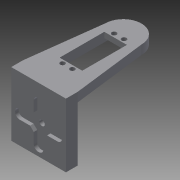
# Autodesk Inventor part: FrontUpperLegShoulder
Saved by Autodesk Inventor 2014 SP1 (Build 180222100, 222)
## iProperties
Created: 2013-09-20
Part Number: FrontUpperLegShoulder
Material: Generic
Document SubType Name: Modeling
Designer: Medrimonia
Density: 1 g/cm^3
Appearance: Default
FrontUpperLegShoulderWidth: 30,000 mm
Author: Medrimonia
Autodesk Inventor part; units mm, degrees
ref_plane "YZ Plane" through (0, 0, 0) normal (1, 0, 0) x (0, 1, 0)
ref_plane "XZ Plane" through (0, 0, 0) normal (0, 1, 0) x (-1, 0, 0)
ref_plane "XY Plane" through (0, 0, 0) normal (0, 0, 1) x (1, 0, 0)
sketch "Sketch1" plane through (0, 0, 0) normal (0, 1, 0) x (-1, 0, 0)
  line L0 (-15, -15) -> (15, -15)
  line L1 (15, -15) -> (15, 15)
  line L2 (15, 15) -> (-15, 15)
  line L3 (-15, 15) -> (-15, -15)
  line L4 (-15, -15) -> (15, 15) construction
  line L5 (15, -15) -> (-15, 15) construction
  line L6 (-2.45, -12.65) -> (2.45, -12.65) construction
  line L7 (2.45, -12.65) -> (2.45, 12.65) construction
  line L8 (2.45, 12.65) -> (-2.45, 12.65) construction
  line L9 (-2.45, 12.65) -> (-2.45, -12.65) construction
  line L10 (-2.45, -12.65) -> (2.45, 12.65) construction
  line L11 (2.45, -12.65) -> (-2.45, 12.65) construction
  line L12 (-12.65, -2.45) -> (12.65, -2.45) construction
  line L13 (12.65, -2.45) -> (12.65, 2.45) construction
  line L14 (12.65, 2.45) -> (-12.65, 2.45) construction
  line L15 (-12.65, 2.45) -> (-12.65, -2.45) construction
  line L16 (-12.65, -2.45) -> (12.65, 2.45) construction
  line L17 (12.65, -2.45) -> (-12.65, 2.45) construction
  line L18 (-12.85, -2.65) -> (12.85, -2.65)
  line L19 (12.85, -2.65) -> (12.85, 2.65)
  line L20 (12.85, 2.65) -> (-12.85, 2.65)
  line L21 (-12.85, 2.65) -> (-12.85, -2.65)
  line L22 (-12.85, -2.65) -> (12.85, 2.65) construction
  line L23 (12.85, -2.65) -> (-12.85, 2.65) construction
  line L24 (-2.65, -12.85) -> (2.65, -12.85)
  line L25 (2.65, -12.85) -> (2.65, 12.85)
  line L26 (2.65, 12.85) -> (-2.65, 12.85)
  line L27 (-2.65, 12.85) -> (-2.65, -12.85)
  line L28 (-2.65, -12.85) -> (2.65, 12.85) construction
  line L29 (2.65, -12.85) -> (-2.65, 12.85) construction
  point P0 (0, 0)
  point P1 (0, 0)
  dimension "d0" = 30
  dimension "d1" = 4.9
  dimension "d2" = 10.2
  dimension "d3" = 0.2
  dimension "d4" = 0.2
  constraints: 60 end point, 12 midpoint, 10 parallel, 10 perpendicular, 5 horizontal
  measures "d0" distance of L1.end L2.end
  measures "d1" distance of L14.end L12.start
  measures "d2" distance between parallel lines of L13 L7
  measures "d3" distance between parallel lines of L25 L7
  measures "d4" distance between parallel lines of L26 L8
extrude "Extrusion1" add sketch "Sketch1" along normal blind 1.9
sketch "Sketch2" plane through (0, 1.9, 0) normal (0, 1, 0) x (1, 0, 0)
  line L0 (15, 15) -> (-15, 15) projected
  line L1 (-15, 15) -> (-15, -15) projected
  line L2 (-15, -15) -> (15, -15) projected
  line L3 (15, -15) -> (15, 15) projected
  circle A0 centre (0, 0) radius 1.5
  dimension "d7" = 3
  constraints: 1 centre point, 1 coincident
  measures "d7" diameter of A0
extrude "Extrusion2" add sketch "Sketch2" along normal blind 2
sketch "Sketch3" plane through (0, 3.9, 0) normal (0, 1, 0) x (1, 0, 0)
  circle A0 centre (0, 0) radius 1.5 projected
  line L0 (15, 15) -> (-15, 15) projected
  line L1 (-15, 15) -> (-15, -15) projected
  line L2 (-15, -15) -> (15, -15) projected
  line L3 (15, -15) -> (15, 15) projected
  circle A1 centre (0, 0) radius 2.75
  dimension "d10" = 5.5
  constraints: 1 centre point, 1 coincident
  measures "d10" diameter of A1
extrude "Extrusion3" add sketch "Sketch3" along normal blind 2.5 contours L3 L2 L1 L0
chamfer "Chamfer1" distance 2 angle 45 1 edges at (-2.65, 0.95, -2.65)
fillet "Fillet1" radius 2.45 1 edges at (-12.85, 0.95, -2.65)
fillet "Fillet2" radius 2.45 1 edges at (-2.65, 0.95, -12.85)
chamfer "Chamfer2" distance 2 angle 45 1 edges at (2.65, 0.95, -2.65)
chamfer "Chamfer3" distance 2 angle 45 1 edges at (2.65, 0.95, 2.65)
fillet "Fillet3" radius 2.45 1 edges at (12.85, 0.95, -2.65)
fillet "Fillet4" radius 2.45 1 edges at (2.65, 0.95, -12.85)
fillet "Fillet5" radius 2.45 1 edges at (12.85, 0.95, 2.65)
fillet "Fillet6" radius 2.45 1 edges at (2.65, 0.95, 12.85)
chamfer "Chamfer4" distance 2 angle 45 1 edges at (-2.65, 0.95, 2.65)
fillet "Fillet7" radius 2.45 2 edges at (-2.65, 0.95, 12.85) (-12.85, 0.95, 2.65)
sketch "Sketch8" plane through (-15, 0, 15) normal (0, 0, 1) x (1, 0, 0)
  line L0 (0, 0) -> (30, 0) projected
  line L1 (30, 0) -> (30, 6.4) projected
  line L2 (0, 6.4) -> (30, 6.4) projected
  line L3 (0, 0) -> (0, 6.4) projected
  line L4 (15, 0) -> (15, 120) construction
  line L5 (30, 6.4) -> (25, 46.4)
  line L6 (25, 46.4) -> (5, 46.4)
  line L7 (5, 46.4) -> (0, 6.4)
  arc A0 (25, 46.4) -> (5, 46.4) centre (15, 46.4) ccw
  dimension "d101" = 40
  dimension "d102" = 20
  constraints: 8 end point, 2 point on circle, 1 centre point, 1 midpoint, 1 perpendicular, 1 other
  measures "d101" distance between parallel lines of L2 L6
  measures "d102" distance of L5.end L6.end
extrude "Extrusion7" add sketch "Sketch8" along normal blind 5
sketch "Sketch9" plane through (-15, 0, 20) normal (0, 0, 1) x (1, 0, 0)
  line L0 (0, 0) -> (30, 0) projected
  line L1 (9.3, 41.75) -> (20.7, 41.75) construction
  line L2 (20.7, 41.75) -> (20.7, 18.25) construction
  line L3 (20.7, 18.25) -> (9.3, 18.25) construction
  line L4 (9.3, 18.25) -> (9.3, 41.75) construction
  line L5 (15, 90) -> (15, 15.8225) construction
  line L6 (9.3, 41.75) -> (9.3, 46.15) construction
  line L7 (9.3, 46.15) -> (20.7, 46.15) construction
  line L8 (20.7, 46.15) -> (20.7, 41.75) construction
  line L9 (20.7, 18.25) -> (20.7, 13.85) construction
  line L10 (20.7, 13.85) -> (9.3, 13.85) construction
  line L11 (9.3, 13.85) -> (9.3, 18.25) construction
  circle A0 centre (12.3, 44.15) radius 1.3
  circle A1 centre (17.7, 44.15) radius 1.3
  line L12 (-17.4512, 30) -> (18.2205, 30) construction
  circle A2 centre (12.3, 15.85) radius 1.3
  circle A3 centre (17.7, 15.85) radius 1.3
  line L13 (8.8, 42.25) -> (21.2, 42.25)
  line L14 (21.2, 42.25) -> (21.2, 17.75)
  line L15 (21.2, 17.75) -> (8.8, 17.75)
  line L16 (8.8, 17.75) -> (8.8, 42.25)
  line L17 (15, 0) -> (15, 83.8502) construction
  dimension "d105" = 11.4
  dimension "d106" = 23.5
  dimension "d107" = 3
  dimension "d108" = 2.4
  dimension "d109" = 4.4
  dimension "d110" = 0.5
  dimension "d111" = 0.5
  dimension "d113" = 2.6
  dimension "d122" = 30
  constraints: 34 end point, 8 parallel, 5 perpendicular, 4 centre point, 3 symmetric about line, 2 collinear, 2 horizontal, 1 point on line, 8 other
  measures "d105" distance between parallel lines of L2 L4
  measures "d106" distance between parallel lines of L3 L1
  measures "d107" distance from line of L6 A0.centre
  measures "d108" distance from line of A3.centre L3
  measures "d109" distance between parallel lines of L1 L7
  measures "d110" distance between parallel lines of L1 L13
  measures "d111" distance between parallel lines of L2 L14
  measures "d113" diameter of A1
  measures "d122" distance between parallel lines of L0 L12
extrude "Extrusion8" cut sketch "Sketch9" against normal through all
sketch "Sketch10" plane through (-15, 0, 20) normal (0, 0, 1) x (1, 0, 0)
  circle A0 centre (17.7, 15.85) radius 1.3 projected
  circle A1 centre (17.7, 44.15) radius 1.3 projected
  circle A2 centre (12.3, 44.15) radius 1.3 projected
  circle A3 centre (12.3, 15.85) radius 1.3 projected
  line L0 (8.8, 17.75) -> (8.8, 42.25) projected
  line L1 (8.8, 42.25) -> (21.2, 42.25) projected
  line L2 (21.2, 42.25) -> (21.2, 17.75) projected
  line L3 (21.2, 17.75) -> (8.8, 17.75) projected
  line L4 (0, 0) -> (30, 0) projected
  line L5 (9.3, 41.75) -> (20.7, 41.75) construction
  line L6 (20.7, 41.75) -> (20.7, 18.25) construction
  line L7 (20.7, 18.25) -> (9.3, 18.25) construction
  line L8 (9.3, 18.25) -> (9.3, 41.75) construction
  line L9 (15, 87.388) -> (15, -76.2197) construction
  line L10 (9.3, 41.75) -> (9.3, 46.15) construction
  line L11 (9.3, 46.15) -> (20.7, 46.15) construction
  line L12 (20.7, 46.15) -> (20.7, 41.75) construction
  line L13 (20.7, 18.25) -> (20.7, 13.85) construction
  line L14 (20.7, 13.85) -> (9.3, 13.85) construction
  line L15 (9.3, 13.85) -> (9.3, 18.25) construction
  line L16 (0.832, 30) -> (29.7617, 30) construction
  line L17 (8.8, 46.65) -> (21.2, 46.65)
  line L18 (21.2, 46.65) -> (21.2, 13.35)
  line L19 (21.2, 13.35) -> (8.8, 13.35)
  line L20 (8.8, 13.35) -> (8.8, 46.65)
  line L21 (15, 0) -> (15, 87.4766) construction
  dimension "d125" = 11.4
  dimension "d126" = 23.5
  dimension "d127" = 4.4
  dimension "d128" = 0.5
  dimension "d130" = 0.5
  dimension "d136" = 30
  constraints: 34 end point, 10 parallel, 5 perpendicular, 2 collinear, 2 horizontal, 1 coincident, 5 other
  measures "d125" distance between parallel lines of L6 L8
  measures "d126" distance between parallel lines of L7 L5
  measures "d127" distance between parallel lines of L5 L11
  measures "d128" distance between parallel lines of L6 L18
  measures "d130" distance between parallel lines of L11 L17
  measures "d136" distance between parallel lines of L4 L16
ref_plane "Work Plane2" through (-15, 0, 17) normal (0, 0, 1) x (1, 0, 0)
extrude "Extrusion10" cut sketch "Sketch10" along normal up to surface (2 mm away) from surface at -5 contours L3 L18 L19 L20 | L20 L17 L18 L1
equation "\"d0\" = FrontUpperLegShoulderWidth"
equation "\"d1\" = ServoArmWidth"
equation "\"d2\" = ServoArmLength"
equation "\"d3\" = ServoArmSpacing"
equation "\"d4\" = ServoArmSpacing"
equation "\"d5\" = ServoArmThickness"
equation "\"d7\" = ServoArmHoleRequired"
equation "\"d8\" = MinimalThickness"
equation "\"d10\" = ServoArmHeadScrewTrace"
equation "\"d11\" = ServoArmHeadScrewThickness"
equation "\"d13\" = ServoArmInternFillet"
equation "\"d16\" = ServoArmExternFillet"
equation "\"d17\" = ServoArmExternFillet"
equation "\"d18\" = ServoArmInternFillet"
equation "\"d21\" = ServoArmInternFillet"
equation "\"d24\" = ServoArmExternFillet"
equation "\"d25\" = ServoArmExternFillet"
equation "\"d26\" = ServoArmExternFillet"
equation "\"d27\" = ServoArmExternFillet"
equation "\"d28\" = ServoArmInternFillet"
equation "\"d31\" = ServoArmExternFillet"
equation "\"d101\" = FrontShoulderHeight"
equation "\"d102\" = FrontShoulderWidth"
equation "\"d103\" = FrontShoulderThickness"
equation "\"d105\" = ServoCoreWidth"
equation "\"d106\" = ServoCoreLength"
equation "\"d107\" = ServoEdgeToFixation"
equation "\"d108\" = ServoCoreToFixation"
equation "\"d109\" = ServoFixationLength"
equation "\"d110\" = ServoTraceSpacing"
equation "\"d111\" = ServoTraceSpacing"
equation "\"d113\" = ServoScrewDiameterRequired"
equation "\"d122\" = FrontShoulderServoCenterDistance"
equation "\"d123\" = FrontShoulderThickness"
equation "\"d125\" = ServoCoreWidth"
equation "\"d126\" = ServoCoreLength"
equation "\"d127\" = ServoFixationLength"
equation "\"d128\" = ServoTraceSpacing"
equation "\"d130\" = ServoTraceSpacing"
equation "\"d136\" = FrontShoulderServoCenterDistance"
equation "\"ServoTraceSpacing\" = 0.5"
equation "\"FrontUpperLegShoulderWidth\" = 30"
equation "\"LegServoThickness\" = 3"
equation "\"FrontShoulderHeight\" = 40"
equation "\"FrontShoulderWidth\" = 20"
equation "\"FrontShoulderThickness\" = 5"
equation "\"FrontShoulderServoCenterDistance\" = 30"
equation "\"d140\" = -LegServoThickness"
equation "\"ServoArmWidth\" = 4.9"
equation "\"ServoArmLength\" = 10.2"
equation "\"ServoArmSpacing\" = 0.2"
equation "\"ServoArmThickness\" = 1.9"
equation "\"ServoArmHoleRequired\" = 3"
equation "\"MinimalThickness\" = 2"
equation "\"ServoArmHeadScrewTrace\" = 5.5"
equation "\"ServoArmHeadScrewThickness\" = 2.5"
equation "\"ServoArmInternFillet\" = 2"
equation "\"ServoArmExternFillet\" = 2.45"
equation "\"ServoCoreWidth\" = 11.4"
equation "\"ServoCoreLength\" = 23.5"
equation "\"ServoEdgeToFixation\" = 3"
equation "\"ServoCoreToFixation\" = 2.4"
equation "\"ServoFixationLength\" = 4.4"
equation "\"ServoScrewDiameterRequired\" = 2.6"
body "Solid1"
